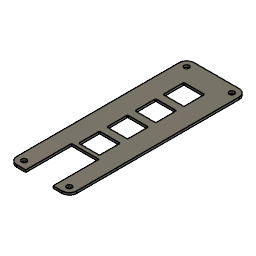
Top (Autodesk Fusion 360 design; units mm, degrees)
part number: 2026-01-31-18-18-28-498
Autodesk Fusion 360 part; units mm, degrees
sketch "Sketch1" plane through (0, 1.51, 0) normal (0, 1, 0) x (-1, 0, 0)
  line L0 (-6.5, 26.325) -> (6.5, 26.325)
  line L1 (-6.5, 12.325) -> (6.5, 12.325)
  line L2 (-7, 25.825) -> (-7, 12.825)
  line L3 (7, 25.825) -> (7, 12.825)
  arc A0 (-6.5, 26.325) -> (-7, 25.825) centre (-6.5, 25.825) ccw
  arc A1 (7, 25.825) -> (6.5, 26.325) centre (6.5, 25.825) ccw
  arc A2 (-7, 12.825) -> (-6.5, 12.325) centre (-6.5, 12.825) ccw
  arc A3 (6.5, 12.325) -> (7, 12.825) centre (6.5, 12.825) ccw
  line L4 (-6.5, 7.275) -> (6.5, 7.275)
  line L5 (-6.5, -6.725) -> (6.5, -6.725)
  line L6 (-7, 6.775) -> (-7, -6.225)
  line L7 (7, 6.775) -> (7, -6.225)
  arc A4 (-6.5, 7.275) -> (-7, 6.775) centre (-6.5, 6.775) ccw
  arc A5 (7, 6.775) -> (6.5, 7.275) centre (6.5, 6.775) ccw
  arc A6 (-7, -6.225) -> (-6.5, -6.725) centre (-6.5, -6.225) ccw
  arc A7 (6.5, -6.725) -> (7, -6.225) centre (6.5, -6.225) ccw
  line L8 (-6.5, -11.775) -> (6.5, -11.775)
  line L9 (-6.5, -25.775) -> (6.5, -25.775)
  line L10 (-7, -12.275) -> (-7, -25.275)
  line L11 (7, -12.275) -> (7, -25.275)
  arc A8 (-6.5, -11.775) -> (-7, -12.275) centre (-6.5, -12.275) ccw
  arc A9 (7, -12.275) -> (6.5, -11.775) centre (6.5, -12.275) ccw
  arc A10 (-7, -25.275) -> (-6.5, -25.775) centre (-6.5, -25.275) ccw
  arc A11 (6.5, -25.775) -> (7, -25.275) centre (6.5, -25.275) ccw
  line L12 (-6.5, -30.825) -> (6.5, -30.825)
  line L13 (-6.5, -44.825) -> (6.5, -44.825)
  line L14 (-7, -31.325) -> (-7, -44.325)
  line L15 (7, -31.325) -> (7, -44.325)
  arc A12 (-6.5, -30.825) -> (-7, -31.325) centre (-6.5, -31.325) ccw
  arc A13 (7, -31.325) -> (6.5, -30.825) centre (6.5, -31.325) ccw
  arc A14 (-7, -44.325) -> (-6.5, -44.825) centre (-6.5, -44.325) ccw
  arc A15 (6.5, -44.825) -> (7, -44.325) centre (6.5, -44.325) ccw
  line L16 (-20.3, -60.027) -> (20.3, -60.027)
  line L17 (20.3, -60.027) -> (20.3, 60.027)
  line L18 (20.3, 60.027) -> (-20.3, 60.027)
  line L19 (-20.3, 60.027) -> (-20.3, -60.027)
  circle A16 centre (-15.3, -55.027) radius 1.7
  circle A17 centre (15.3, -55.027) radius 1.7
  circle A18 centre (15.3, 55.027) radius 1.7
  circle A19 centre (-15.3, 55.027) radius 1.7
  line L20 (-9.25, 60.027) -> (9.25, 60.027)
  line L21 (9.25, 60.027) -> (9.25, 29.027)
  line L22 (9.25, 29.027) -> (-9.25, 29.027)
  line L23 (-9.25, 29.027) -> (-9.25, 60.027)
  dimension "d4" = 3.4
  dimension "d5" = 3.4
  dimension "d6" = 3.4
  dimension "d7" = 3.4
  dimension "d8" = 5
  dimension "d9" = 5
  dimension "d10" = 5
  dimension "d11" = 5
  dimension "d12" = 5
  dimension "d13" = 5
  dimension "d14" = 5
  dimension "d15" = 5
  dimension "d16" = 11.05
  dimension "d17" = 18.5
  dimension "d18" = 31
  constraint horizontal L20
  constraint vertical L21
  constraint horizontal L22
  constraint vertical L23
  measures "d4" diameter of A16
  measures "d5" diameter of A17
  measures "d6" diameter of A18
  measures "d7" diameter of A19
  measures "d8" distance of L18 A19.centre
  measures "d9" distance of L19 A19.centre
  measures "d10" distance of L18 A18.centre
  measures "d11" distance of L17 A18.centre
  measures "d12" distance of L17 A17.centre
  measures "d13" distance of L16 A17.centre
  measures "d14" distance of L19 A16.centre
  measures "d15" distance of L16 A16.centre
  measures "d16" distance of L18.end L20.start
  measures "d17" distance of L20.start L20.end
  measures "d18" distance of L20.start L22.end
extrude "Extrude1" add sketch "Sketch1" along normal blind 1.5 contours L16 L17 L18 L19 L21 L22 L23
fillet "Fillet1" radius 5 4 edges at (-20.3, 2.26, -60.027) (20.3, 2.26, -60.027) (20.3, 2.26, 60.027) (-20.3, 2.26, 60.027)
move_body "Move1" bodies 1 to x (1, 0, 0) y (0, 1, 0) z (0, 0, 1) at (0, 3.5, 0)
move_body "Move2" bodies 1 to x (1, 0, 0) y (0, 1, 0) z (0, 0, 1) at (0, -5, 0)
equation "d16 = 10 mm + 1.4 mm - 0.35 mm"
